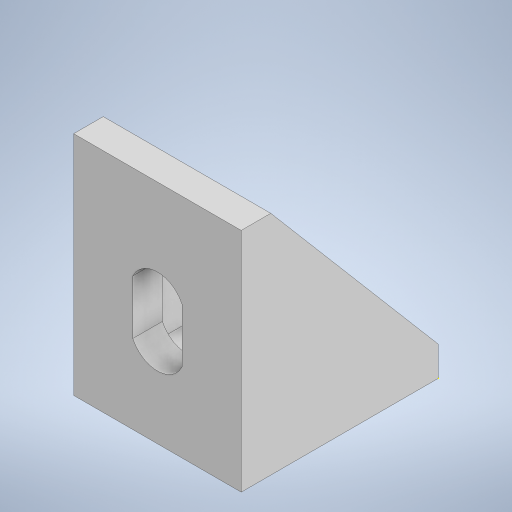
# Autodesk Inventor part: 90 Degree attachment T Slot
Saved by Autodesk Inventor 2023.5 (Build 275446000, 446)
## iProperties
Created: 2024-08-12
Part Number: 90 Degree attachment T Slot
Material: Generic
Document SubType Name: Modeling
Designer: punny
Density: 1 g/cm^3
Appearance: Default
Author: punny
Autodesk Inventor part; units mm, degrees
ref_plane "YZ Plane" through (0, 0, 0) normal (1, 0, 0) x (0, 1, 0)
ref_plane "XZ Plane" through (0, 0, 0) normal (0, 1, 0) x (-1, 0, 0)
ref_plane "XY Plane" through (0, 0, 0) normal (0, 0, 1) x (1, 0, 0)
sketch "Sketch1" plane through (0, 0, 0) normal (0, 0, 1) x (1, 0, 0)
  line L0 (0, 0) -> (0, 3)
  line L1 (0, 3) -> (17, 3)
  line L2 (17, 3) -> (17, 0)
  line L3 (17, 0) -> (0, 0)
  dimension "d0" = 3
  dimension "d1" = 17
  constraints: 8 end point, 3 perpendicular, 1 vertical
  measures "d0" distance of L0.start L0.end
  measures "d1" distance of L0.end L1.end
extrude "Extrusion1" add sketch "Sketch1" along normal blind 20
sketch "Sketch2" plane through (17, 0, 0) normal (1, 0, 0) x (0, 0, -1)
  point P0 (0, 0)
sketch "Sketch3" plane through (0, 3, 0) normal (0, 1, 0) x (1, 0, 0)
  line L0 (17, -20) -> (17, -17)
  line L1 (17, 0) -> (17, -20) projected
  line L2 (17, -17) -> (0, -17)
  line L3 (0, 0) -> (0, -20) projected
  line L4 (17, -20) -> (0, -20) projected
  line L5 (0, -20) -> (0, -17)
  line L6 (0, -20) -> (17, -20)
  dimension "d4" = 3
  constraints: 8 end point, 2 perpendicular, 2 point on line, 1 horizontal
  measures "d4" distance of L0.start L0.end
extrude "Extrusion2" add sketch "Sketch3" along normal blind 20
sketch "Sketch4" plane through (17, 0, 0) normal (1, 0, 0) x (0, 0, -1)
  line L0 (-20, 23) -> (-17, 23) projected
  line L1 (0, 3) -> (-17, 23)
  line L2 (0, 3) -> (-17, 3) projected
  line L3 (-17, 23) -> (-17, 3)
  line L4 (-17, 3) -> (0, 3)
  point P0 (0, 0)
  constraints: 6 end point, 2 perpendicular
extrude "Extrusion3" add sketch "Sketch4" against normal blind 2.4
sketch "Sketch5" plane through (0, 0, 0) normal (-1, 0, 0) x (0, 0, 1)
  line L0 (17, 3) -> (17, 23) projected
  line L1 (0, 3) -> (0, 0) projected
  line L2 (17, 23) -> (0, 3)
  line L3 (0, 3) -> (17, 3)
  line L4 (17, 23) -> (0, 3) projected
  line L5 (17, 3) -> (17, 23)
  constraints: 6 end point, 2 perpendicular
extrude "Extrusion4" add sketch "Sketch5" against normal blind 2.4
sketch "Sketch6" plane through (14.6, 3, 17) normal (0, 0, -1) x (-1, 0, 0)
  line L0 (-2.4, -3) -> (-2.4, 20) projected
  line L1 (-2.4, -3) -> (6.1, -3)
  line L2 (14.6, -3) -> (-2.4, -3) projected
  line L3 (6.1, 5) -> (6.7519, 5)
  line L4 (6.7519, 10.5) -> (6.1, 10.5)
  line L5 (6.1, 10.5) -> (3.6, 10.5)
  line L6 (3.6, 10.5) -> (8.6, 10.5)
  line L7 (6.1, 5) -> (3.6, 5)
  line L8 (3.6, 5) -> (8.6, 5)
  line L9 (8.6, 5) -> (8.6, 10.5)
  line L10 (3.6, 10.5) -> (3.6, 5)
  arc A0 (8.6, 10.5) -> (3.6, 10.5) centre (6.1, 9.3544) ccw
  arc A1 (3.6, 5) -> (8.6, 5) centre (6.1, 6.1456) ccw
  dimension "d11" = 8.5
  constraints: 18 end point, 4 point on circle, 3 point on line, 2 centre point, 1 horizontal, 1 midpoint
  measures "d11" distance of L0.start L1.end
extrude "Extrusion5" cut sketch "Sketch6" against normal through all
sketch "Sketch7" plane through (2.4, 3, 17) normal (0, 1, 0) x (1, 0, 0)
  line L0 (-2.4, -3) -> (-2.4, 20)
  line L1 (-2.4, -3) -> (6.1, -3)
  line L2 (14.6, -3) -> (-2.4, -3)
  line L3 (6.1, 5) -> (6.7519, 5)
  line L4 (6.7519, 10.5) -> (6.1, 10.5)
  line L5 (6.1, 10.5) -> (3.6, 10.5)
  line L6 (3.6, 10.5) -> (8.6, 10.5)
  line L7 (6.1, 5) -> (3.6, 5)
  line L8 (3.6, 5) -> (8.6, 5)
  line L9 (8.6, 5) -> (8.6, 10.5)
  line L10 (3.6, 10.5) -> (3.6, 5)
  arc A0 (8.6, 10.5) -> (3.6, 10.5) centre (6.1, 9.3544) ccw
  arc A1 (3.6, 5) -> (8.6, 5) centre (6.1, 6.1456) ccw
  dimension "d25" = 8.5
  constraints: 22 end point, 4 point on circle, 3 point on line, 2 centre point, 1 horizontal, 1 midpoint
  measures "d25" distance of L0.start L1.end
extrude "Extrusion6" cut sketch "Sketch7" against normal through all
body "Solid1"
